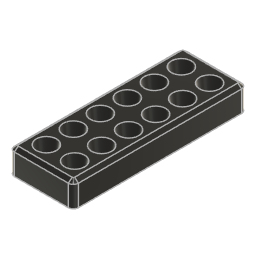
ER16-Collet-Insert (Autodesk Fusion 360 design; units mm, degrees)
Autodesk Fusion 360 part; units mm, degrees
sketch "sketch 521" plane through (0, 0, 0) normal (0, 0, 1) x (-1, 0, 0)
  arc A0 (-4, -134.9) -> (-0.1, -131) centre (-4, -131) ccw
  line L0 (-0.1, -131) -> (-0.1, -4)
  arc A1 (-0.1, -4) -> (-4, -0.1) centre (-4, -4) ccw
  line L1 (-4, -0.1) -> (-46, -0.1)
  arc A2 (-46, -0.1) -> (-49.9, -4) centre (-46, -4) ccw
  line L2 (-49.9, -4) -> (-49.9, -131)
  arc A3 (-49.9, -131) -> (-46, -134.9) centre (-46, -131) ccw
  line L3 (-46, -134.9) -> (-4, -134.9)
extrude "Extrude1" add sketch "sketch 521" along normal blind 19
sketch "sketch 464" plane through (0, 0, 0) normal (0, 0, 1) x (-1, 0, 0)
  circle A0 centre (-14, -36) radius 7.85
  circle A1 centre (-14, -78) radius 7.85
  circle A2 centre (-14, -120) radius 7.85
  circle A3 centre (-36, -99) radius 7.85
  circle A4 centre (-36, -57) radius 7.85
  circle A5 centre (-36, -15) radius 7.85
  circle A6 centre (-36, -36) radius 7.85
  circle A7 centre (-36, -78) radius 7.85
  circle A8 centre (-36, -120) radius 7.85
  circle A9 centre (-14, -99) radius 7.85
  circle A10 centre (-14, -57) radius 7.85
  circle A11 centre (-14, -15) radius 7.85
extrude "Extrude2" cut sketch "sketch 464" against normal blind 14 draft -7.9 from surface at 19
chamfer "Chamfer1" distance 3 distance2 2.5 8 edges at (49.9, 67.5, 19) (48.7577, 133.7577, 19) (25, 134.9, 19) (1.2423, 133.7577, 19) (0.1, 67.5, 19) (1.2423, 1.2423, 19) (25, 0.1, 19) (48.7577, 1.2423, 19) measured on face at (28.0844, 132.4844, 19) measured on face at (28.0844, 132.4844, 19) measured on face at (28.0844, 132.4844, 19) measured on face at (28.0844, 132.4844, 19) measured on face at (28.0844, 132.4844, 19) measured on face at (28.0844, 132.4844, 19) measured on face at (28.0844, 132.4844, 19) measured on face at (28.0844, 132.4844, 19)
